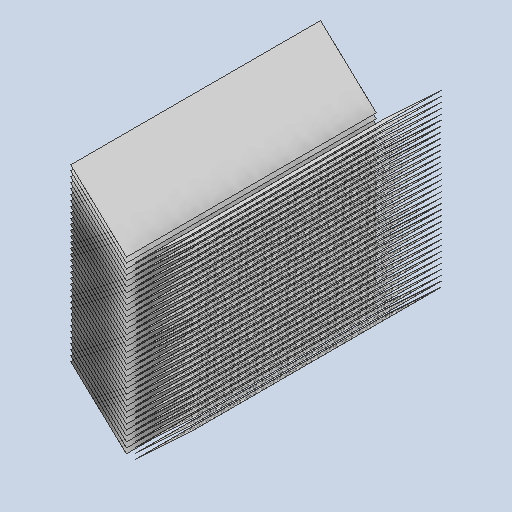
# Autodesk Inventor part: МОО 0101 лист жабра
Saved by Autodesk Inventor 2024.2 (Build 282272000, 272)
## iProperties
Created: 2024-06-15
Part Number: МОО 0101 лист жабра
Material: Stainless Steel
Document SubType Name: Sheet Metal
Designer: pokla
Density: 8 g/cm^3
Sheet Metal Rule: Default_mm
Appearance: Default
Stock Number: МОО 0101 лист жабра
Author: pokla
Autodesk Inventor part; units mm, degrees
ref_plane "YZ Plane" through (0, 0, 0) normal (1, 0, 0) x (0, 1, 0)
ref_plane "XZ Plane" through (0, 0, 0) normal (0, 1, 0) x (-1, 0, 0)
ref_plane "XY Plane" through (0, 0, 0) normal (0, 0, 1) x (1, 0, 0)
sketch "Sketch1" plane through (0, 0, 0) normal (0, 0, 1) x (1, 0, 0)
  line L0 (-750, 0) -> (750, 0) construction
  line L1 (750, 0) -> (750, -2100) construction
  line L2 (750, -2100) -> (110, -2700) construction
  line L3 (110, -2700) -> (-110, -2700) construction
  line L4 (-110, -2700) -> (-750, -2100) construction
  line L5 (-750, -2100) -> (-750, 0) construction
  line L6 (-725, -40) -> (725, -40) construction
  line L7 (-725, -2089.1692) -> (-100.1138, -2675) construction
  line L8 (-100.1138, -2675) -> (100.1138, -2675) construction
  line L9 (100.1138, -2675) -> (725, -2089.1692) construction
  line L10 (0, -2700) -> (0, 0) construction
  line L11 (55, -2700) -> (55, 0) construction
  line L12 (-55, -2700) -> (-55, 0) construction
  line L13 (725, -2089.1692) -> (725, -40) construction
  line L14 (-725, -40) -> (-725, -2089.1692) construction
  line L15 (725, -40) -> (55, -664.7851)
  point P0 (0, -40)
  dimension "d0" = 1500
  dimension "d2" = 220
  dimension "d3" = 600
  dimension "d5" = 2700
  dimension "d7" = 40
  dimension "d10" = 1450
  dimension "d11" = 25
  dimension "d13" = 55
  dimension "d14" = 55
  dimension "d16" = 133
  measures "d0" distance of L0.start L0.end
  measures "d2" distance of L2.end L3.end
  measures "d3" vertical distance of L2.end L1.end
  measures "d5" distance between parallel lines of L0 L3
  measures "d7" distance between parallel lines of L0 L6
  measures "d10" distance of L6.end L6.start
  measures "d11" distance between parallel lines of L3 L8
  measures "d13" distance between parallel lines of L10 L11
  measures "d14" distance between parallel lines of L10 L12
  measures "d16" angle of L13 L15
contour flange "Contour Flange1" sketch "Sketch1" thickness 0.8 bend radius 0.8 width 3000 along (0, 0, -1) mid plane no both sides no wall seen from (390, -352.3926, 0) lies toward (0.6819984, -0.7313537, 0) curves L15
bend "Bend1"
corner "Corner1"
pattern_linear "Rectangular Pattern1" count 34 spacing 62 along (0, -1, 0) of "Contour Flange1"
mirror "Mirror1" about plane through (0, 0, 0) normal (1, 0, 0) of "Contour Flange1", "Rectangular Pattern1"
equation "\"d14\" = d13"
equation "\"d17\" = Thickness"
equation "\"d18\" = BendReliefWidth"
equation "\"d19\" = BendReliefDepth"
equation "\"d20\" = MinimumRemnant"
equation "\"d21\" = TransitionRadius"
equation "\"d23\" = BendRadius"
equation "\"d25\" = CornerReliefSize"
equation "\"d26\" = GapSize"
equation "\"d27\" = JacobiRadiusSize"
equation "\"BendRadius\" = Thickness"
equation "\"BendReliefWidth\" = Thickness"
equation "\"BendReliefDepth\" = 0.5 * Thickness"
equation "\"CornerReliefSize\" = 4 * Thickness"
equation "\"MinimumRemnant\" = 2 * Thickness"
equation "\"TransitionRadius\" = BendRadius"
equation "\"JacobiRadiusSize\" = BendRadius"
equation "\"GapSize\" = Thickness"
equation "\"Thickness\" = 0.8"
body "Solid1"
